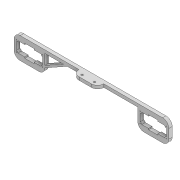
# Autodesk Inventor part: UltrasonicHolder
Saved by Autodesk Inventor 2022 (Build 260153000, 153)
## iProperties
Created: 2023-02-15
Part Number: UltrasonicHolder
Material: Generic
Document SubType Name: Modeling
Designer: MVeszpremi
Density: 1 g/cm^3
Appearance: Default
Author: MVeszpremi
Autodesk Inventor part; units mm, degrees
ref_plane "YZ Plane" through (0, 0, 0) normal (1, 0, 0) x (0, 1, 0)
ref_plane "XZ Plane" through (0, 0, 0) normal (0, 1, 0) x (-1, 0, 0)
ref_plane "XY Plane" through (0, 0, 0) normal (0, 0, 1) x (1, 0, 0)
sketch "Sketch1" plane through (0, 0, 0) normal (0, 0, 1) x (1, 0, 0)
  line L0 (0, 0) -> (250, 0)
  line L1 (250, 0) -> (250, 35)
  line L2 (250, 35) -> (0, 35)
  line L3 (0, 35) -> (0, 0)
  line L4 (25, 35) -> (25, 0)
  line L5 (3.9, 8.9) -> (46.1, 8.9)
  line L6 (46.1, 8.9) -> (46.1, 26.1)
  line L7 (46.1, 26.1) -> (3.9, 26.1)
  line L8 (3.9, 26.1) -> (3.9, 8.9)
  line L9 (3.9, 8.9) -> (46.1, 26.1) construction
  line L10 (46.1, 8.9) -> (3.9, 26.1) construction
  circle A0 centre (3.9, 26.1) radius 2.5
  circle A1 centre (46.1, 26.1) radius 2.5
  circle A2 centre (3.9, 8.9) radius 2.5
  circle A3 centre (46.1, 8.9) radius 2.5
  circle A4 centre (3.9, 26.1) radius 0.6
  circle A5 centre (46.1, 26.1) radius 0.6
  circle A6 centre (3.9, 8.9) radius 0.6
  circle A7 centre (46.1, 8.9) radius 0.6
  line L11 (125, 35) -> (125, 0)
  line L12 (225, 35) -> (225, 0)
  line L13 (246.1, 8.9) -> (203.9, 8.9)
  line L14 (203.9, 8.9) -> (203.9, 26.1)
  line L15 (203.9, 26.1) -> (246.1, 26.1)
  line L16 (246.1, 26.1) -> (246.1, 8.9)
  line L17 (246.1, 8.9) -> (203.9, 26.1) construction
  line L18 (203.9, 8.9) -> (246.1, 26.1) construction
  circle A8 centre (246.1, 26.1) radius 2.5
  circle A9 centre (203.9, 26.1) radius 2.5
  circle A10 centre (246.1, 8.9) radius 2.5
  circle A11 centre (203.9, 8.9) radius 2.5
  circle A12 centre (246.1, 26.1) radius 0.6
  circle A13 centre (203.9, 26.1) radius 0.6
  circle A14 centre (246.1, 8.9) radius 0.6
  circle A15 centre (203.9, 8.9) radius 0.6
  line L19 (17.5, 7) -> (32.5, 7)
  line L20 (32.5, 7) -> (32.5, 28)
  line L21 (32.5, 28) -> (17.5, 28)
  line L22 (17.5, 28) -> (17.5, 7)
  line L23 (17.5, 7) -> (32.5, 28) construction
  line L24 (32.5, 7) -> (17.5, 28) construction
  line L25 (46.1, 26.1) -> (3.9, 26.1)
  line L26 (232.5, 7) -> (217.5, 7)
  line L27 (217.5, 7) -> (217.5, 28)
  line L28 (217.5, 28) -> (232.5, 28)
  line L29 (232.5, 28) -> (232.5, 7)
  point P0 (25, 17.5)
  point P1 (225, 17.5)
  point P2 (6.4, 26.1)
  point P3 (17.5, 26.1)
  point P4 (32.5, 26.1)
  point P5 (43.6, 26.1)
  point P6 (46.1, 23.6)
  point P7 (46.1, 11.4)
  point P8 (43.6, 8.9)
  point P9 (32.5, 8.9)
  point P10 (17.5, 8.9)
  point P11 (6.4, 8.9)
  point P12 (3.9, 11.4)
  point P13 (3.9, 23.6)
  point P14 (217.5, 8.9)
  point P15 (206.4, 8.9)
  point P16 (203.9, 11.4)
  point P17 (203.9, 23.6)
  point P18 (206.4, 26.1)
  point P19 (217.5, 26.1)
  point P20 (232.5, 26.1)
  point P21 (243.6, 26.1)
  point P22 (246.1, 23.6)
  point P23 (246.1, 11.4)
  point P24 (243.6, 8.9)
  point P25 (232.5, 8.9)
  dimension "d0" = 250
  dimension "d1" = 35
  dimension "d2" = 17.2
  dimension "d3" = 42.2
  dimension "d4" = 5
  dimension "d5" = 5
  dimension "d6" = 5
  dimension "d7" = 5
  dimension "d8" = 1.2
  dimension "d9" = 1.2
  dimension "d10" = 1.2
  dimension "d11" = 1.2
  dimension "d12" = 25
  dimension "d13" = 15
  dimension "d14" = 21
  constraints: 60 end point, 19 symmetric about line, 16 centre point, 16 coincident, 9 midpoint, 6 parallel, 4 perpendicular, 3 horizontal, 2 point on line, 8 other
  measures "d0" distance of L1.end L2.end
  measures "d1" distance of L0.end L1.end
  measures "d2" distance of L5.end L6.end
  measures "d3" distance of L6.end L7.end
  measures "d4" diameter of A0
  measures "d5" diameter of A1
  measures "d6" diameter of A2
  measures "d7" diameter of A3
  measures "d8" diameter of A4
  measures "d9" diameter of A5
  measures "d10" diameter of A6
  measures "d11" diameter of A7
  measures "d12" distance between parallel lines of L3 L4
  measures "d13" distance of L20.end L21.end
  measures "d14" distance of L19.end L20.end
extrude "Extrusion1" add sketch "Sketch1" along normal blind 5.5 contours L3 L2 L4 L21 L22 L7 A0 L8 A2 L5 L19 L0 | L4 L19 L20 L5 A3 L6 A1 L7 L21 L2 L11 L0 | L11 L2 L12 L28 L27 L15 A9 L14 A11 L13 L26 L0 | L12 L26 L29 L13 A10 L16 A8 L15 L28 L2 L1 L0 | A2 L8 A6 L5 | L5 A6 L8 A2 | A3 L6 A7 L5 | L5 A7 L6 A3 | A1 L6 A5 L7 | L7 A5 L6 A1 | A0 L8 A4 L7 | L7 A4 L8 A0 | A6 L8 L5 | L5 L8 A6 | A7 L6 L5 | L5 L6 A7 | A10 L16 A14 L13 | L13 A14 L16 A10 | A11 L14 A15 L13 | L13 A15 L14 A11 | A5 L6 L7 | L7 L6 A5 | A4 L8 L7 | L7 L8 A4 | A9 L14 A13 L15 | L15 A13 L14 A9 | A8 L16 A12 L15 | L15 A12 L16 A8 | A14 L16 L13 | L13 L16 A14 | A15 L14 L13 | L13 L14 A15 | A13 L14 L15 | L15 L14 A13 | A12 L16 L15 | L15 L16 A12
extrude "Extrusion2" cut sketch "Sketch1" along normal blind 5.5 contours A6 L8 L5 | L5 L8 A6 | A7 L6 L5 | L5 L6 A7 | A5 L6 L7 | L7 L6 A5 | A4 L8 L7 | L7 L8 A4 | A14 L16 L13 | L13 L16 A14 | A15 L14 L13 | L13 L14 A15 | A13 L14 L15 | L15 L14 A13 | A12 L16 L15 | L15 L16 A12
sketch "Sketch2" plane through (0, 0, 5.5) normal (0, 0, 1) x (1, 0, 0)
  line L0 (200, -30) -> (50, -30)
  line L1 (50, -30) -> (50, 30)
  line L2 (50, 30) -> (200, 30)
  line L3 (200, 30) -> (200, -30)
  line L4 (0, 0) -> (250, 0) projected
  line L5 (200, -30) -> (50, 30) construction
  line L6 (50, -30) -> (200, 30) construction
  point P0 (125, 0)
  point P1 (50, 0)
  point P2 (200, 0)
  dimension "d19" = 150
  dimension "d20" = 60
  constraints: 12 end point, 3 midpoint, 2 parallel, 1 horizontal, 1 perpendicular
  measures "d19" distance of L1.end L2.end
  measures "d20" distance of L0.end L1.end
extrude "Extrusion3" cut sketch "Sketch2" against normal blind 5.5 contours L4 L1 L2 L3
sketch "Sketch3" plane through (0, 0, 5.5) normal (0, 0, 1) x (1, 0, 0)
  line L0 (50, 30) -> (200, 30) projected
  line L1 (105, 30) -> (145, 30)
  line L2 (145, 30) -> (145, 35)
  line L3 (145, 35) -> (105, 35)
  line L4 (105, 35) -> (105, 30)
  point P0 (0, 0)
  point P1 (145, 30)
  dimension "d23" = 40
  dimension "d24" = 5
  dimension "d25" = 55
  constraints: 8 end point, 2 parallel, 1 horizontal, 1 perpendicular, 1 point on line
  measures "d23" distance of L2.end L3.end
  measures "d24" distance of L3.end L1.start
  measures "d25" distance of L0.start L1.start
extrude "Extrusion4" add sketch "Sketch3" along normal blind 10
sketch "Sketch4" plane through (105, 35, 5.5) normal (0, 1, 0) x (-1, 0, 0)
  line L0 (0, 10) -> (-40, 10) projected
  line L1 (-20, 10) -> (-20, 0)
  line L2 (-145, 0) -> (105, 0) projected
  circle A0 centre (-10, 5) radius 1.5
  circle A1 centre (-30, 5) radius 1.5
  line L3 (-10, 5) -> (-30, 5)
  point P0 (105, -5.5)
  dimension "d28" = 10
  dimension "d29" = 3
  dimension "d30" = 3
  dimension "d31" = 10
  constraints: 4 end point, 2 centre point, 2 midpoint, 1 horizontal
  measures "d28" distance from line of L1 L3.start
  measures "d29" diameter of A0
  measures "d30" diameter of A1
  measures "d31" distance from line of L1 L3.end
extrude "Extrusion5" cut sketch "Sketch4" against normal blind 10
fillet "Fillet1" radius 10 8 edges at (0, 35, 2.75) (50, 0, 2.75) (0, 0, 2.75) (145, 32.5, 15.5) (105, 32.5, 15.5) (200, 0, 2.75) (250, 0, 2.75) (250, 35, 2.75)
sketch "Sketch5" plane through (0, 0, 5.5) normal (0, 0, 1) x (1, 0, 0)
  arc A0 (40, 0) -> (50, 10) centre (40, 10) ccw projected
  line L0 (50, 10) -> (86.2042, 30)
  line L1 (50, 30) -> (105, 30) projected
  line L2 (50, 10) -> (50, 30) projected
  line L3 (50, 13.4273) -> (80, 30)
  arc A1 (0, 10) -> (10, 0) centre (10, 10) ccw projected
  line L4 (10, 0) -> (40, 0) projected
  arc A2 (40, 0) -> (50, 10) centre (40, 10) ccw projected
  line L5 (50, 10) -> (50, 30) projected
  line L6 (50, 30) -> (105, 30) projected
  line L7 (105, 30) -> (105, 35) projected
  line L8 (105, 35) -> (10, 35) projected
  arc A3 (10, 35) -> (0, 25) centre (10, 25) ccw projected
  line L9 (0, 25) -> (0, 10) projected
  circle A4 centre (46.1, 8.9) radius 0.6 projected
  circle A5 centre (3.9, 8.9) radius 0.6 projected
  circle A6 centre (46.1, 26.1) radius 0.6 projected
  circle A7 centre (3.9, 26.1) radius 0.6 projected
  line L10 (6.4, 26.1) -> (17.5, 26.1) projected
  line L11 (17.5, 26.1) -> (17.5, 28) projected
  line L12 (17.5, 28) -> (32.5, 28) projected
  line L13 (32.5, 28) -> (32.5, 26.1) projected
  line L14 (32.5, 26.1) -> (43.6, 26.1) projected
  arc A8 (43.6, 26.1) -> (46.1, 23.6) centre (46.1, 26.1) ccw projected
  line L15 (46.1, 23.6) -> (46.1, 11.4) projected
  arc A9 (46.1, 11.4) -> (43.6, 8.9) centre (46.1, 8.9) ccw projected
  line L16 (43.6, 8.9) -> (32.5, 8.9) projected
  line L17 (32.5, 8.9) -> (32.5, 7) projected
  line L18 (32.5, 7) -> (17.5, 7) projected
  line L19 (17.5, 7) -> (17.5, 8.9) projected
  line L20 (17.5, 8.9) -> (6.4, 8.9) projected
  arc A10 (6.4, 8.9) -> (3.9, 11.4) centre (3.9, 8.9) ccw projected
  line L21 (3.9, 11.4) -> (3.9, 23.6) projected
  arc A11 (3.9, 23.6) -> (6.4, 26.1) centre (3.9, 26.1) ccw projected
  point P0 (0, 0)
  dimension "d35" = 3
  dimension "d36" = 30
  constraints: 4 end point, 3 point on line, 1 parallel
  measures "d35" distance between parallel lines of L0 L3
  measures "d36" distance of L1.start L3.end
extrude "Extrusion6" add sketch "Sketch5" against normal blind 5.5 contours L2 L3 L1 L0
body "Solid1"
